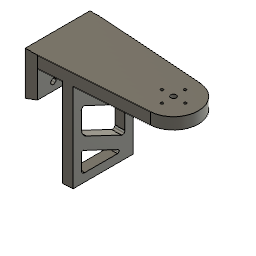
Femur 1 (Autodesk Fusion 360 design; units mm, degrees)
Autodesk Fusion 360 part; units mm, degrees
note: some values were not read from the file. Set by a fixed rule: which sketch regions a step uses.
sketch "Sketch1" plane through (0, 0, 0) normal (0, 1, 0) x (1, 0, 0)
  line L0 (3.75, -19.5) -> (-3.75, -19.5)
  line L1 (-3.75, -19.5) -> (-3.75, 19.5)
  line L2 (-3.75, 19.5) -> (3.75, 19.5)
  line L3 (3.75, 19.5) -> (3.75, -19.5)
  line L4 (3.75, -19.5) -> (-3.75, 19.5) construction
  line L5 (-3.75, -19.5) -> (3.75, 19.5) construction
  circle A0 centre (66.05, 0) radius 15
  line L6 (3.75, -19.5) -> (67.1215, -14.9617)
  line L7 (3.75, 19.5) -> (67.1215, 14.9617)
  dimension "d1" = 7.5
  dimension "d2" = 39
  dimension "d4" = 30
  constraint horizontal L0
  constraint perpendicular L0 L1
  constraint parallel L0 L2
  constraint parallel L1 L3
  constraint coincident L4 origin
  constraint coincident L5 origin
  constraint tangent A0 L7
  constraint tangent A0 L6
  constraint coincident A0 L7.end
  constraint coincident A0 L6.end
  measures "d1" distance of L1.end L2.end
  measures "d2" distance of L0.end L1.end
  measures "d4" diameter of A0
extrude "Extrude1" add sketch "Sketch1" along normal blind 7
sketch "Sketch2" plane through (0, 7, 0) normal (0, 1, 0) x (-1, 0, 0)
  line L0 (-3.75, 19.5) -> (-67.1215, 14.9617)
  arc A0 (-67.1215, 14.9617) -> (-67.1215, -14.9617) centre (-66.05, 0) ccw
  line L1 (-67.1215, -14.9617) -> (-3.75, -19.5)
  line L2 (-3.75, -19.5) -> (3.75, -19.5)
  line L3 (3.75, -19.5) -> (3.75, 19.5)
  line L4 (3.75, 19.5) -> (-3.75, 19.5)
  line L5 (3.75, -19.5) -> (-3.75, -19.5)
  line L6 (-3.75, -19.5) -> (-3.75, 19.5)
  line L7 (-3.75, 19.5) -> (3.75, 19.5)
  line L8 (3.75, 19.5) -> (3.75, -19.5)
  constraint horizontal L5
  constraint vertical L6
  constraint horizontal L7
  constraint vertical L8
  constraint coincident L0.start L4.end
  constraint coincident L2.end L3.start
extrude "Extrude2" add sketch "Sketch2" against normal blind 23.35 contours L2 L3 L4 L5 L6 L7 L8
sketch "Sketch3" plane through (0, 0, -19.5) normal (0, 0, -1) x (-1, 0, 0)
  line L0 (3.75, -16.35) -> (3.75, 7)
  line L1 (3.75, 7) -> (-3.75, 7)
  line L2 (-3.75, 7) -> (-3.75, 0)
  line L3 (-3.75, 0) -> (-3.75, -16.35)
  line L4 (-3.75, -16.35) -> (3.75, -16.35)
  line L5 (3.75, -16.35) -> (3.75, -19.22)
  line L6 (3.75, -19.22) -> (-3.75, -16.35)
  dimension "d9" = 2.87
  constraint coincident L0.start L4.end
  constraint perpendicular L4 L5
  constraint coincident L3.end L4.start
  measures "d9" distance of L0.start L5.end
extrude "Extrude3" add sketch "Sketch3" against normal blind 39 contours L4 L5 L6
sketch "Sketch4" plane through (0, 0, 0) normal (0, -1, 0) x (1, 0, 0)
  line L0 (3.75, 19.5) -> (3.75, -19.5)
  line L1 (3.75, -19.5) -> (67.1215, -14.9617)
  arc A0 (67.1215, -14.9617) -> (67.1215, 14.9617) centre (66.05, 0) ccw
  line L2 (67.1215, 14.9617) -> (3.75, 19.5)
  line L3 (3.75, -19.5) -> (17.7142, -18.5)
  line L4 (17.7142, -18.5) -> (23.6989, -18.0714)
  line L5 (3.75, 19.5) -> (17.7142, 18.5)
  line L6 (17.7142, 18.5) -> (23.6989, 18.0714)
  line L7 (23.6989, 18.0714) -> (23.6989, -18.0714)
  line L8 (17.7142, 18.5) -> (17.7142, -18.5)
  dimension "d12" = 14
  dimension "d13" = 6
  dimension "d14" = 14
  dimension "d15" = 6
  constraint coincident L0.end L1.start
  constraint parallel L1 L3
  constraint parallel L1 L4
  constraint coincident L0.start L2.end
  constraint parallel L2 L5
  constraint parallel L2 L6
  measures "d12" distance of L0.end L3.end
  measures "d13" distance of L3.end L4.end
  measures "d14" distance of L0.start L5.end
  measures "d15" distance of L5.end L6.end
extrude "Extrude4" add sketch "Sketch4" along normal blind 53.35 contours L1 L2 L4 L6 L7 L8
sketch "Sketch5" plane through (23.6989, 0, 0) normal (1, 0, 0) x (0, 0, -1)
  line L0 (18.0714, 0) -> (-18.0714, 0)
  line L1 (-18.0714, 0) -> (-18.0714, -53.35)
  line L2 (-18.0714, -53.35) -> (18.0714, -53.35)
  line L3 (18.0714, -53.35) -> (18.0714, 0)
  line L4 (-11.0714, -48.35) -> (8.6618, -48.35)
  line L5 (11.0714, -5) -> (-8.6618, -5)
  line L6 (13.0714, -7) -> (13.0714, -17.5)
  line L7 (11.64, -16.8156) -> (-9.0931, -6.9022)
  line L8 (-13.0714, -46.35) -> (-13.0714, -35.85)
  line L9 (9.0931, -46.4478) -> (-11.64, -36.5344)
  line L10 (10.9243, -39.8234) -> (-10.2282, -29.7094)
  line L11 (-10.9243, -13.5266) -> (10.2282, -23.6406)
  line L12 (13.0714, -38.4701) -> (13.0714, -28.1514)
  line L13 (13.0714, -15.9134) -> (13.0714, -5)
  line L14 (-13.0714, -14.8799) -> (-13.0714, -25.1986)
  line L15 (-13.0714, -37.4366) -> (-13.0714, -48.35)
  arc A0 (8.6618, -48.35) -> (9.0931, -46.4478) centre (8.6618, -47.35) ccw
  arc A1 (-11.64, -36.5344) -> (-13.0714, -37.4366) centre (-12.0714, -37.4366) ccw
  arc A2 (11.64, -16.8156) -> (13.0714, -15.9134) centre (12.0714, -15.9134) ccw
  arc A3 (-8.6618, -5) -> (-9.0931, -6.9022) centre (-8.6618, -6) ccw
  arc A4 (13.0714, -7) -> (11.0714, -5) centre (11.0714, -7) ccw
  arc A5 (-13.0714, -46.35) -> (-11.0714, -48.35) centre (-11.0714, -46.35) ccw
  arc A6 (10.9243, -39.8234) -> (13.0714, -38.4701) centre (11.5714, -38.4701) ccw
  arc A7 (-10.9243, -13.5266) -> (-13.0714, -14.8799) centre (-11.5714, -14.8799) ccw
  arc A8 (13.0714, -28.1514) -> (10.2282, -23.6406) centre (8.0714, -28.1514) ccw
  arc A9 (-13.0714, -25.1986) -> (-10.2282, -29.7094) centre (-8.0714, -25.1986) ccw
  point P0 (-13.0714, -5)
  point P1 (13.0714, -48.35)
  point P2 (13.0714, -25)
  point P3 (-13.0714, -28.35)
  point P4 (13.0714, -40.85)
  point P5 (-13.0714, -12.5)
  dimension "d19" = 12.5
  dimension "d20" = 7.5
  dimension "d21" = 12.5
  dimension "d22" = 7.5
  dimension "d23" = 7.5
  dimension "d24" = 7.5
  dimension "d25" = 1
  dimension "d26" = 2
  dimension "d27" = 1.5
  dimension "d28" = 5
  constraint perpendicular L5 L6
  constraint collinear L12 L13
  constraint collinear L14 L15
  constraint coincident P1 L4
  constraint coincident P1 L9
  constraint tangent L4 A0
  constraint tangent L9 A0
  constraint coincident L8.end L15
  constraint coincident L8.end L9
  constraint tangent L15 A1
  constraint tangent L9 A1
  constraint equal A0 A1
  constraint coincident L6.end L7
  constraint tangent L13 A2
  constraint tangent L7 A2
  constraint equal A0 A2
  constraint coincident P0 L7
  constraint coincident P0 L5
  constraint tangent L7 A3
  constraint tangent L5 A3
  constraint equal A0 A3
  constraint coincident L13.end L6
  constraint coincident L13.end L5
  constraint tangent L6 A4
  constraint tangent L5 A4
  constraint coincident L15.end L4
  constraint coincident L15.end L8
  constraint tangent L4 A5
  constraint tangent L8 A5
  constraint equal A4 A5
  constraint coincident P4 L10
  constraint coincident P4 L12
  constraint tangent L10 A6
  constraint tangent L12 A6
  constraint coincident P5 L11
  constraint coincident P5 L14
  constraint tangent L11 A7
  constraint tangent L14 A7
  constraint equal A6 A7
  constraint coincident P2 L12
  constraint coincident P2 L11
  constraint tangent L12 A8
  constraint tangent L11 A8
  constraint coincident P3 L10
  constraint coincident P3 L14
  constraint tangent L10 A9
  constraint tangent L14 A9
  constraint equal A8 A9
  measures "d19" distance of L13.end L6.end
  measures "d20" distance of L6.end P2
  measures "d21" distance of L15.end L8.end
  measures "d22" distance of L8.end P3
  measures "d23" distance of P1 P4
  measures "d24" distance of P0 P5
  measures "d25" radius of A0
  measures "d26" radius of A4
  measures "d27" radius of A6
  measures "d28" radius of A8
extrude "Extrude5" cut sketch "Sketch5" against normal blind 9 contours L4 L8 L9 L15 A0 A1 A5 | L5 L6 L7 L13 A2 A3 A4 | L10 L11 L12 L14 A6 A7 A8 A9
sketch "Sketch6" plane through (0, 0, 0) normal (0, -1, 0) x (1, 0, 0)
  line L0 (23.6989, 18.0714) -> (23.6989, -18.0714)
  line L1 (23.6989, -18.0714) -> (67.1215, -14.9617)
  arc A0 (67.1215, -14.9617) -> (67.1215, 14.9617) centre (66.05, 0) ccw
  line L2 (67.1215, 14.9617) -> (23.6989, 18.0714)
  circle A1 centre (66.05, 0) radius 10.35
  dimension "d31" = 20.7
  constraint concentric A0 A1
  measures "d31" diameter of A1
extrude "Extrude6" cut sketch "Sketch6" against normal blind 1.6 contours A1
sketch "Sketch7" plane through (0, 1.6, 0) normal (0, -1, 0) x (1, 0, 0)
  circle A0 centre (66.05, 0) radius 10.35
  circle A1 centre (66.05, 0) radius 1.6
  line L0 (66.05, 0) -> (59.05, 0)
  line L1 (66.05, 0) -> (73.05, 0)
  line L2 (66.05, 0) -> (66.05, -7)
  line L3 (66.05, 0) -> (66.05, 7)
  circle A2 centre (59.05, 0) radius 0.75
  circle A3 centre (66.05, 7) radius 0.75
  circle A4 centre (73.05, 0) radius 0.75
  circle A5 centre (66.05, -7) radius 0.75
  dimension "d34" = 3.2
  dimension "d35" = 7
  dimension "d36" = 7
  dimension "d37" = 7
  dimension "d38" = 7
  dimension "d39" = 1.5
  dimension "d40" = 1.5
  dimension "d41" = 1.5
  dimension "d42" = 1.5
  constraint concentric A0 A1
  constraint coincident A0.centre A1.centre
  constraint horizontal L0
  constraint parallel L0 L1
  constraint perpendicular L1 L2
  constraint perpendicular L1 L3
  constraint coincident L0.end A2.centre
  constraint coincident L3.end A3.centre
  constraint coincident L1.end A4.centre
  constraint coincident L2.end A5.centre
  measures "d34" diameter of A1
  measures "d35" distance of A0.centre L0.end
  measures "d36" distance of A0.centre L1.end
  measures "d37" distance of A0.centre L2.end
  measures "d38" distance of A0.centre L3.end
  measures "d39" diameter of A2
  measures "d40" diameter of A3
  measures "d41" diameter of A4
  measures "d42" diameter of A5
extrude "Extrude7" cut sketch "Sketch7" against normal blind 13 contours A1 L1 L3 | A1 L1 L2 | A1 L0 L3 | A1 L0 L2 | A2 | A3 | A4 | A5
sketch "Sketch8" plane through (3.75, 0, 0) normal (1, 0, 0) x (0, 0, -1)
  line L0 (19.5, 0) -> (-19.5, 0)
  line L1 (-19.5, 0) -> (-19.5, -16.35)
  line L2 (-19.5, -16.35) -> (19.5, -16.35)
  line L3 (19.5, -16.35) -> (19.5, 0)
  line L4 (19.5, -16.35) -> (10, -16.35)
  line L5 (10, -16.35) -> (10, -11.35)
  circle A0 centre (10, -11.35) radius 1.6
  line L6 (10, -11.35) -> (-10, -11.35)
  circle A1 centre (-10, -11.35) radius 1.6
  dimension "d45" = 9.5
  dimension "d46" = 5
  dimension "d47" = 3.2
  dimension "d48" = 20
  dimension "d49" = 3.2
  constraint coincident L2.end L3.start
  constraint perpendicular L3 L4
  constraint perpendicular L4 L5
  constraint coincident L5.end A0.centre
  constraint perpendicular L5 L6
  constraint coincident L6.end A1.centre
  measures "d45" distance of L2.end L4.end
  measures "d46" distance of L4.end L5.end
  measures "d47" diameter of A0
  measures "d48" distance of L5.end L6.end
  measures "d49" diameter of A1
extrude "Extrude8" cut sketch "Sketch8" against normal blind 19 contours L5 A0 L6 | L5 A0 L6 | A1
sketch "Sketch9" plane through (0, -53.35, 0) normal (0, -1, 0) x (1, 0, 0)
  line L0 (23.6989, 18.0714) -> (17.7142, 18.5)
  line L1 (17.7142, 18.5) -> (17.7142, -18.5)
  line L2 (17.7142, -18.5) -> (23.6989, -18.0714)
  line L3 (23.6989, -18.0714) -> (23.6989, 18.0714)
  circle A0 centre (20.7416, 0) radius 1.6
  circle A1 centre (20.7416, 10) radius 1.6
  circle A2 centre (20.7416, -10) radius 1.6
  dimension "d52" = 3.2
  dimension "d53" = 10
  dimension "d54" = 10
  dimension "d55" = 3.2
  dimension "d56" = 3.2
  measures "d52" diameter of A0
  measures "d53" distance of A0.centre A2.centre
  measures "d54" distance of A0.centre A1.centre
  measures "d55" diameter of A1
  measures "d56" diameter of A2
extrude "Extrude9" cut sketch "Sketch9" against normal blind 4 contours A0 | A1 | A2
